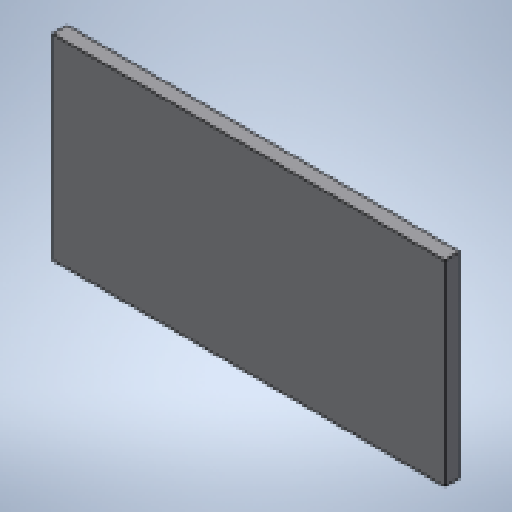
# Autodesk Inventor part: base1
Saved by Autodesk Inventor 2023 (Build 270158000, 158)
## iProperties
Created: 2022-09-27
Part Number: base1
Material: Generic
Document SubType Name: Modeling
Designer: kleber
Density: 1 g/cm^3
Appearance: Default
Author: kleber
Autodesk Inventor part; units mm, degrees
ref_plane "YZ Plane" through (0, 0, 0) normal (1, 0, 0) x (0, 1, 0)
ref_plane "XZ Plane" through (0, 0, 0) normal (0, 1, 0) x (-1, 0, 0)
ref_plane "XY Plane" through (0, 0, 0) normal (0, 0, 1) x (1, 0, 0)
sketch "Sketch1" plane through (0, 0, 0) normal (0, 0, 1) x (1, 0, 0)
  line L0 (25.75, -50.425) -> (115.75, -50.425)
  line L1 (115.75, -50.425) -> (-284.25, -50.425)
  line L2 (-284.25, -50.425) -> (-284.25, 149.575)
  line L3 (-284.25, 149.575) -> (115.75, 149.575)
  line L4 (115.75, 149.575) -> (115.75, -50.425)
  point P0 (0, 0)
  dimension "d2" = 90
  dimension "d3" = 400
  dimension "d4" = 200
  constraints: 10 end point, 2 parallel, 1 horizontal, 1 perpendicular
  measures "d2" distance of L0.start L0.end
  measures "d3" distance of L2.end L3.end
  measures "d4" distance of L1.end L2.end
extrude "Extrusion1" add sketch "Sketch1" along normal blind 15
body "Solid1"
